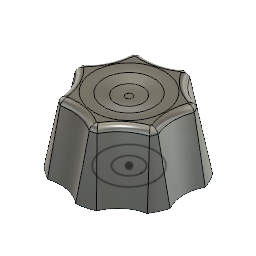
knob v5 (Autodesk Fusion 360 design; units mm, degrees)
Autodesk Fusion 360 part; units mm, degrees
sketch "Sketch1" plane through (0, 0, 0) normal (0, 1, 0) x (1, 0, 0)
  circle A0 centre (0, 0) radius 15
  circle A1 centre (13.6368, 17.9706) radius 9.3906
  circle A2 centre (-5.5475, 21.8662) radius 9.3906
  circle A3 centre (-20.5545, 9.2961) radius 9.3906
  circle A4 centre (-20.0835, -10.2741) radius 9.3906
  circle A5 centre (-4.4892, -22.1077) radius 9.3906
  circle A6 centre (14.4855, -17.2938) radius 9.3906
  circle A7 centre (22.5524, 0.5428) radius 9.3906
  dimension "d1" = 30
  dimension "d3" = 360
  constraint coincident A0.centre origin
  measures "d1" diameter of A0
extrude "Extrude1" add sketch "Sketch1" along normal blind 16 draft -10 contours A0 A1 A2 A3 A4 A5 A6 A7
fillet "Fillet1" radius 1.5 14 edges at (6.6441, 16, 7.9321) (2.9949, 16, 11.8048) (-2.0591, 16, 10.1401) (-7.362, 16, 9.7017) (-9.2117, 16, 4.7124) (-12.1752, 16, 0.293) (-9.4277, 16, -4.2638) (-7.8202, 16, -9.3363) (-2.5445, 16, -10.0293) (2.4236, 16, -11.9352) (6.2548, 16, -8.2426) (10.8424, 16, -5.5466) (10.3441, 16, -0.249) (11.0967, 16, 5.0186)
sketch "Sketch2" plane through (0, 16, 0) normal (0, 1, 0) x (-1, 0, 0)
  arc A0 (6.9002, -8.4638) -> (-2.0308, -10.7296) centre (5.5475, -21.8662) ccw
  arc A1 (6.9002, -8.4638) -> (7.1226, -8.2776) centre (0, 0) ccw
  arc A2 (10.9195, 0.1177) -> (7.1226, -8.2776) centre (20.5545, -9.2961) ccw
  arc A3 (10.9195, 0.1177) -> (10.9125, 0.4077) centre (0, 0) ccw
  arc A4 (6.7161, 8.6106) -> (10.9125, 0.4077) centre (20.0835, 10.2741) ccw
  arc A5 (6.7161, 8.6106) -> (6.4851, 8.7859) centre (0, 0) ccw
  arc A6 (-2.5446, 10.6195) -> (6.4851, 8.7859) centre (4.4892, 22.1077) ccw
  arc A7 (-2.5446, 10.6195) -> (-2.8257, 10.5482) centre (0, 0) ccw
  arc A8 (-9.8892, 4.6317) -> (-2.8257, 10.5482) centre (-14.4855, 17.2938) ccw
  arc A9 (-9.8892, 4.6317) -> (-10.0087, 4.3675) centre (0, 0) ccw
  arc A10 (-9.787, -4.8439) -> (-10.0087, 4.3675) centre (-22.5524, -0.5428) ccw
  arc A11 (-9.787, -4.8439) -> (-9.6549, -5.1021) centre (0, 0) ccw
  arc A12 (-2.315, -10.6719) -> (-9.6549, -5.1021) centre (-13.6368, -17.9706) ccw
  arc A13 (-2.315, -10.6719) -> (-2.0308, -10.7296) centre (0, 0) ccw
  circle A14 centre (0, 0) radius 7.5
  dimension "d9" = 15
  constraint concentric A1 A14
  measures "d9" diameter of A14
extrude "Extrude2" cut sketch "Sketch2" against normal blind 0.942 draft -80 contours A14
fillet "Fillet2" radius 15 2 edges at (6.9925, 16, 2.7121) (2.0116, 15.058, -0.7802)
sketch "Sketch3" plane through (0, 0, 0) normal (0, -1, 0) x (1, 0, 0)
  arc A0 (5.7471, 13.8554) -> (1.5532, 14.9194) centre (0, 0) ccw
  arc A1 (-7.2493, 13.1319) -> (1.5532, 14.9194) centre (-4.4892, 22.1077) ccw
  arc A2 (-7.2493, 13.1319) -> (-10.696, 10.5164) centre (0, 0) ccw
  arc A3 (-14.7868, 2.5199) -> (-10.696, 10.5164) centre (-20.0835, 10.2741) ccw
  arc A4 (-14.7868, 2.5199) -> (-14.8909, -1.8056) centre (0, 0) ccw
  arc A5 (-11.1895, -9.9897) -> (-14.8909, -1.8056) centre (-20.5545, -9.2961) ccw
  arc A6 (-11.1895, -9.9897) -> (-7.8727, -12.768) centre (0, 0) ccw
  arc A7 (0.8337, -14.9768) -> (-7.8727, -12.768) centre (-5.5475, -21.8662) ccw
  arc A8 (0.8337, -14.9768) -> (5.0739, -14.1158) centre (0, 0) ccw
  arc A9 (12.2291, -8.6861) -> (5.0739, -14.1158) centre (13.6368, -17.9706) ccw
  arc A10 (12.2291, -8.6861) -> (14.1997, -4.8341) centre (0, 0) ccw
  arc A11 (14.4158, 4.1455) -> (14.1997, -4.8341) centre (22.5524, -0.5428) ccw
  arc A12 (14.4158, 4.1455) -> (12.6328, 8.0877) centre (0, 0) ccw
  arc A13 (5.7471, 13.8554) -> (12.6328, 8.0877) centre (14.4855, 17.2938) ccw
  circle A14 centre (0, 0) radius 6.5
  circle A15 centre (0, 0) radius 3.1
  dimension "d11" = 6.2
  dimension "d14" = 13
  constraint concentric A0 A14
  constraint concentric A14 A15
  measures "d11" diameter of A15
  measures "d14" diameter of A14
extrude "Extrude3" cut sketch "Sketch3" against normal blind 4.0266 draft -40 contours A14 | A15
extrude "Extrude4" cut sketch "Sketch3" against normal blind 13 contours A15
named bodies: "Knob"
